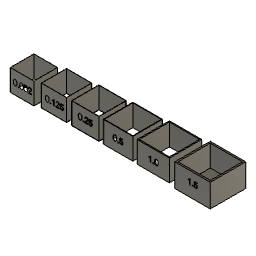
VeggþykktarTest (Autodesk Fusion 360 design; units mm, degrees)
Autodesk Fusion 360 part; units mm, degrees
note: some values were not read from the file. Chosen so that the rebuilt part matches the saved one: which bodies a step acts on; that a step has no effect.
form "Form1" [no effect]
sketch "Sketch1" plane through (0, 0, 0) normal (0, 0, 1) x (1, 0, 0)
  line L0 (0, 0) -> (26.5, 0)
  line L1 (26.5, 0) -> (26.5, 26.5)
  line L2 (26.5, 26.5) -> (0, 26.5)
  line L3 (0, 26.5) -> (0, 0)
  line L4 (-0.5, -0.5) -> (27, -0.5)
  line L5 (27, -0.5) -> (27, 27)
  line L6 (27, 27) -> (-0.5, 27)
  line L7 (-0.5, 27) -> (-0.5, -0.5)
  line L8 (32.5, 0) -> (60.5, 0)
  line L9 (60.5, 0) -> (60.5, 28)
  line L10 (60.5, 28) -> (32.5, 28)
  line L11 (32.5, 28) -> (32.5, 0)
  line L12 (61.5, -1) -> (61.5, 29)
  line L13 (61.5, 29) -> (31.5, 29)
  line L14 (31.5, 29) -> (31.5, -1)
  line L15 (31.5, -1) -> (61.5, -1)
  line L16 (68.5, 0) -> (98.5, 0)
  line L17 (98.5, 0) -> (98.5, 30)
  line L18 (98.5, 30) -> (68.5, 30)
  line L19 (68.5, 30) -> (68.5, 0)
  line L20 (67, -1.5) -> (100, -1.5)
  line L21 (100, -1.5) -> (100, 31.5)
  line L22 (100, 31.5) -> (67, 31.5)
  line L23 (67, 31.5) -> (67, -1.5)
  line L24 (-30, -0.0853) -> (-5, -0.0853)
  line L25 (-5, -0.0853) -> (-5, 24.9147)
  line L26 (-5, 24.9147) -> (-30, 24.9147)
  line L27 (-30, 24.9147) -> (-30, -0.0853)
  line L28 (-30.25, -0.3353) -> (-4.75, -0.3353)
  line L29 (-4.75, -0.3353) -> (-4.75, 25.1647)
  line L30 (-4.75, 25.1647) -> (-30.25, 25.1647)
  line L31 (-30.25, 25.1647) -> (-30.25, -0.3353)
  line L32 (-58.5, 23.3249) -> (-35, 23.3249)
  line L33 (-35, 23.3249) -> (-35, -0.1751)
  line L34 (-35, -0.1751) -> (-58.5, -0.1751)
  line L35 (-58.5, -0.1751) -> (-58.5, 23.3249)
  line L36 (-35.125, -0.0501) -> (-58.375, -0.0501)
  line L37 (-58.375, -0.0501) -> (-58.375, 23.1999)
  line L38 (-58.375, 23.1999) -> (-35.125, 23.1999)
  line L39 (-35.125, 23.1999) -> (-35.125, -0.0501)
  line L40 (-85.5, 19.921) -> (-63.5, 19.921)
  line L41 (-63.5, 19.921) -> (-63.5, -2.079)
  line L42 (-63.5, -2.079) -> (-85.5, -2.079)
  line L43 (-85.5, -2.079) -> (-85.5, 19.921)
  line L44 (-63.5625, -2.0165) -> (-85.4375, -2.0165)
  line L45 (-85.4375, -2.0165) -> (-85.4375, 19.8585)
  line L46 (-85.4375, 19.8585) -> (-63.5625, 19.8585)
  line L47 (-63.5625, 19.8585) -> (-63.5625, -2.0165)
  dimension "d1" = 26.5
  dimension "d2" = 26.5
  dimension "d4" = 28
  dimension "d5" = 1
  dimension "d6" = 30
  dimension "d7" = 30
  dimension "d8" = 1.5
  dimension "d9" = 25
  dimension "d10" = 25
  dimension "d11" = 0.25
  dimension "d12" = 5
  dimension "d13" = 6
  dimension "d14" = 8
  dimension "d27" = 23.5
  dimension "d28" = 23.5
  dimension "d29" = 0.125
  dimension "d30" = 22
  dimension "d31" = 22
  dimension "d32" = 0.0625
  dimension "d33" = 5
  dimension "d34" = 5
  dimension "d43" = 28
  constraint horizontal L0
  constraint vertical L1
  constraint horizontal L2
  constraint vertical L3
  constraint coincident L0.start L3.end
  constraint horizontal L8
  constraint vertical L9
  constraint horizontal L10
  constraint vertical L11
  constraint horizontal L16
  constraint vertical L17
  constraint horizontal L18
  constraint vertical L19
  constraint horizontal L24
  constraint vertical L25
  constraint horizontal L26
  constraint vertical L27
  constraint horizontal L32
  constraint vertical L33
  constraint horizontal L34
  constraint vertical L35
  constraint horizontal L40
  constraint vertical L41
  constraint horizontal L42
  constraint vertical L43
  measures "d1" distance of L0.start L0.end
  measures "d2" distance of L0.start L2.end
  measures "d4" distance of L8.start L8.end
  measures "d6" distance of L16.start L16.end
  measures "d7" distance of L16.start L18.end
  measures "d9" distance of L24.start L24.end
  measures "d10" distance of L24.start L26.end
  measures "d12" distance of L3 L25
  measures "d13" distance of L1 L11
  measures "d14" distance of L9 L19
  measures "d27" distance of L32.start L32.end
  measures "d28" distance of L32.start L34.end
  measures "d30" distance of L40.start L40.end
  measures "d31" distance of L40.start L42.end
  measures "d33" distance of L35 L41
  measures "d34" distance of L27 L33
  measures "d43" distance of L8 L10
extrude "Extrude1" add sketch "Sketch1" along normal blind 20 contours L4 L5 L6 L7 | L12 L13 L14 L15 | L20 L21 L22 L23 | L28 L29 L30 L31 makes body 1 at (-0.5, 17.8333, 6.6667) makes body 2 at (-30.25, 16.6647, 6.6667) makes body 3 at (41.5, -1, 6.6667) makes body 4 at (89, 31.5, 6.6667)
sketch "Sketch2" plane through (0, -0.3353, 0) normal (0, -1, 0) x (1, 0, 0)
  line L0 (-30.25, 0) -> (-4.75, 0)
  line L1 (-4.75, 0) -> (-4.75, 20)
  line L2 (-4.75, 20) -> (-30.25, 20)
  line L3 (-30.25, 20) -> (-30.25, 0)
  line L4 (-24.0522, 6.5243) -> (-10.4773, 6.3206) construction
  line L5 (-10.4773, 6.3206) -> (-10.373, 13.2719) construction
  line L6 (-10.373, 13.2719) -> (-23.9478, 13.4757) construction
  line L7 (-23.9478, 13.4757) -> (-24.0522, 6.5243) construction
  line L8 (8.5093, 6.6279) -> (16.9992, 6.6328) construction
  line L9 (16.9992, 6.6328) -> (16.9956, 12.8297) construction
  line L10 (16.9956, 12.8297) -> (8.5057, 12.8248) construction
  line L11 (8.5057, 12.8248) -> (8.5093, 6.6279) construction
  line L12 (42.2909, 6.1542) -> (49.9915, 6.0611) construction
  line L13 (49.9915, 6.0611) -> (50.0728, 12.7851) construction
  line L14 (50.0728, 12.7851) -> (42.3722, 12.8782) construction
  line L15 (42.3722, 12.8782) -> (42.2909, 6.1542) construction
  line L16 (79.3601, 6.8132) -> (81.0301, 6.8) construction
  line L17 (81.0301, 6.8) -> (81.0825, 13.433) construction
  line L18 (81.0825, 13.433) -> (79.4125, 13.4462) construction
  line L19 (79.4125, 13.4462) -> (79.3601, 6.8132) construction
  dimension "d17" = 5
  dimension "d18" = 5
  dimension "d19" = 5
  dimension "d20" = 5
  text T0 "0.25" font "Arial" height 5 align left top in box 13.5764 x 6.9521 at (-24.0522, 6.5243) x (0.999887, -0.015005) y (0.015005, 0.999887) spacing 1
  text T1 "0.5" font "Arial" height 5 align left top in box 8.49 x 6.1969 at (8.5093, 6.6279) x (1, 0.000583) y (-0.000583, 1) spacing 1
  text T2 "1.0" font "Arial" height 5 align left top in box 7.7011 x 6.7245 at (42.2909, 6.1542) x (0.999927, -0.012092) y (0.012092, 0.999927) spacing 1
  text T3 "1.5" font "Arial" height 5 align left top in box 1.67 x 6.6332 at (79.3601, 6.8132) x (0.999969, -0.007898) y (0.007898, 0.999969) spacing 1
extrude "Extrude2" cut sketch "Sketch2" against normal blind 3 text T0 T1 T2 T3 bodies 1 2 3 4 makes body 5 at (-30.25, 16.6647, 6.6667)
extrude "Extrude3" cut sketch "Sketch2" along normal blind 6 text T1 bodies 1 makes body 6 at (9.8141, 0, 10.6814)
extrude "Extrude4" cut sketch "Sketch2" along normal blind 6 text T2 T3 bodies 3 4 makes body 7 at (49.0077, -1, 10.6537)
extrude "Extrude5" add sketch "Sketch1" along normal blind 20 separate body contours L32 L33 L34 L35 | L40 L41 L42 L43 makes body 8 at (-58.5, 7.6582, 6.6667) makes body 9 at (-78.1667, 19.921, 13.3333)
sketch "Sketch3" plane through (0, -0.1751, 0) normal (0, -1, 0) x (1, 0, 0)
  line L0 (-58.5, 0) -> (-35, 0)
  line L1 (-35, 0) -> (-35, 20)
  line L2 (-35, 20) -> (-58.5, 20)
  line L3 (-58.5, 20) -> (-58.5, 0)
  line L4 (-54.6493, 4.4779) -> (-36.239, 4.5256) construction
  line L5 (-36.239, 4.5256) -> (-36.2597, 12.5263) construction
  line L6 (-36.2597, 12.5263) -> (-54.6701, 12.4786) construction
  line L7 (-54.6701, 12.4786) -> (-54.6493, 4.4779) construction
  line L8 (-82.3946, 3.8512) -> (-77.8741, 3.9645) construction
  line L9 (-77.8741, 3.9645) -> (-78.0913, 12.6295) construction
  line L10 (-78.0913, 12.6295) -> (-82.6118, 12.5161) construction
  line L11 (-82.6118, 12.5161) -> (-82.3946, 3.8512) construction
  dimension "d37" = 5
  dimension "d38" = 5
  text T0 "0.125" font "Arial" height 5 align left top in box 18.4104 x 8.0007 at (-54.6493, 4.4779) x (0.999997, 0.002593) y (-0.002593, 0.999997) spacing 1
  text T1 "0.062" font "Arial" height 5 align left top in box 4.5219 x 8.6677 at (-82.3946, 3.8512) x (0.999686, 0.025066) y (-0.025066, 0.999686) spacing 1
extrude "Extrude6" cut sketch "Sketch3" against normal blind 12 text T0 bodies 8 makes body 10 at (-53.3573, -0.0501, 10.3378)
extrude "Extrude7" cut sketch "Sketch3" along normal blind 4 text T1 bodies 9 makes body 11 at (-81.2513, -2.079, 10.4054) makes body 12 at (-71.2019, -2.0165, 10.1702) makes body 13 at (-75.4277, -2.0165, 10.5515)
extrude "Extrude8" add sketch "Sketch1" against normal blind 1.5 separate body contours L16 L17 L18 L19 makes body 14
extrude "Extrude9" add sketch "Sketch1" against normal blind 1.5 contours L20 L21 L22 L23 bodies 4 14
hidden bodies 2 6 7 10 11 12 13
